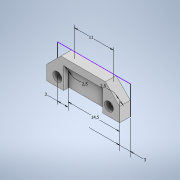
# Autodesk Inventor part: switchholder
Saved by Autodesk Inventor 2022 (Build 260153000, 153)
## iProperties
Created: 2021-01-15
Part Number: switchholder
Material: Generic
Document SubType Name: Modeling
Designer: papa
Density: 1 g/cm^3
Appearance: Default
Author: papa
Autodesk Inventor part; units mm, degrees
ref_plane "YZ Plane" through (0, 0, 0) normal (1, 0, 0) x (0, 1, 0)
ref_plane "XZ Plane" through (0, 0, 0) normal (0, 1, 0) x (-1, 0, 0)
ref_plane "XY Plane" through (0, 0, 0) normal (0, 0, 1) x (1, 0, 0)
sketch "Sketch1" plane through (0, 0, 0) normal (0, 0, 1) x (1, 0, 0)
  line L0 (20.5, 0) -> (20.5, 8)
  line L1 (20.5, 8) -> (0, 8)
  line L2 (0, 8) -> (0, 0)
  circle A0 centre (3, 2.5) radius 1.25
  circle A1 centre (17.5, 2.5) radius 1.25
  line L3 (4.75, 0) -> (15.75, 0)
  line L4 (15.75, 0) -> (15.75, 6)
  line L5 (15.75, 6) -> (4.75, 6)
  line L6 (4.75, 6) -> (4.75, 0)
  line L7 (0, 0) -> (4.75, 0)
  line L8 (15.75, 0) -> (20.5, 0)
  dimension "d0" = 2.5
  dimension "d1" = 2.5
  dimension "d2" = 14.5
  dimension "d7" = 3
  dimension "d8" = 3
  dimension "d9" = 11
  constraints: 18 end point, 5 parallel, 3 horizontal, 3 perpendicular, 2 centre point, 1 collinear
  measures "d0" diameter of A0
  measures "d1" diameter of A1
  measures "d2" distance of A1.centre A0.centre
  measures "d7" distance from line of L2 A0.centre
  measures "d8" distance from line of A1.centre L0
  measures "d9" distance between parallel lines of L4 L6
extrude "Extrusion1" add sketch "Sketch1" along normal blind 3 contours L8 L4 L5 L6 L7 L2 L1 L0
extrude "Extrusion2" add sketch "Sketch1" along normal blind 1.5 contours L3 L6 L5 L4
chamfer "Chamfer1" distance 4 angle 45 2 edges at (0, 8, 1.5) (20.5, 8, 1.5)
chamfer "Chamfer2" distance 1.5 angle 45 2 edges at (1.75, 2.5, 0) (16.25, 2.5, 0)
body "Solid1"
